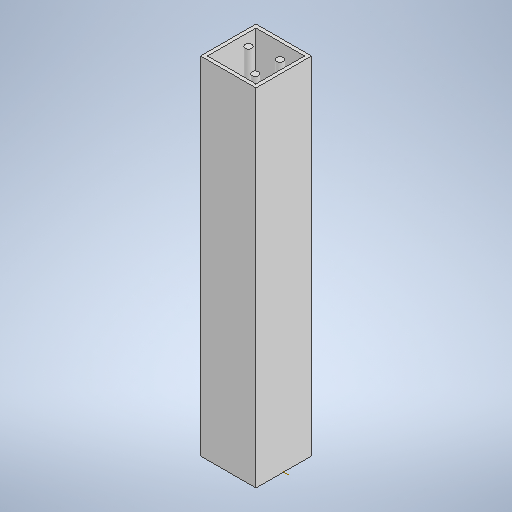
# Autodesk Inventor part: TS_Magazin_int
Saved by Autodesk Inventor 2025.2 (Build 292293000, 293)
## iProperties
Created: 2025-05-27
Part Number: TS_Magazin_int
Material: Generisch
Document SubType Name: Modeling
Designer: tino
Density: 1 g/cm^3
Appearance: Vorgabe
Mass: 3200 g
Surface Area: 1728 cm^2
Volume: 3200 cm^3
Author: tino
Autodesk Inventor part; units mm, degrees
ref_plane "YZ Plane" through (0, 0, 0) normal (1, 0, 0) x (0, 1, 0)
ref_plane "XZ Plane" through (0, 0, 0) normal (0, 1, 0) x (-1, 0, 0)
ref_plane "XY Plane" through (0, 0, 0) normal (0, 0, 1) x (1, 0, 0)
sketch "Skizze1" plane through (0, 0, 0) normal (0, 0, 1) x (1, 0, 0)
  line L0 (-40, 40) -> (40, 40)
  line L1 (40, 40) -> (40, -40)
  line L2 (40, -40) -> (-40, -40)
  line L3 (-40, -40) -> (-40, 40)
  line L4 (-40, 40) -> (40, -40) construction
  line L5 (40, 40) -> (-40, -40) construction
  point P0 (0, 0)
  dimension "d0" = 80
  dimension "d1" = 80
  constraints: 12 end point, 2 midpoint, 2 parallel, 1 horizontal, 1 perpendicular
  measures "d0" distance of L0.start L0.end
  measures "d1" distance of L0.end L1.end
extrude "Extrusion1" add sketch "Skizze1" along normal blind 500
sketch "Skizze2" plane through (0, 0, 500) normal (0, 0, 1) x (1, 0, 0)
  spline S0 degree 3 poles (30.8941, -22.3608) (33.2455, -20.1357) (33.4278, -16.4642) (34.1009, -12.3897) (34.4408, -6.5615) (32.3239, 0.3889) (27.6464, 2.5629) (18.7777, 8.3578) (6.0522, 19.3642) (-10.5837, 24.0919) (-22.9305, 22.7109) (-28.1368, 17.5955) (-28.9312, 16.6042) knots 0 0 0 0 0.05535 0.076528 0.211782 0.295547 0.382964 0.432922 0.754884 0.81234 0.967238 1 1 1 1
  spline S1 degree 3 poles (-28.9312, 16.6042) (-32.363, 12.3217) (-33.9219, 4.96) (-34.2212, -5.2183) (-33.7128, -11.7973) (-30.1787, -16.4552) (-26.4199, -18.3019) (-21.7499, -13.8164) (-22.8916, -9.4321) (-23.5075, -1.7153) (-24.1566, 7.4043) (-16.6489, 14.0721) (-3.6681, 12.4997) (3.1986, 4.5284) (3.2907, 1.6248) (4.5253, 0.0908) (6.4773, -0.7371) (8.3789, 1.0012) (13.1845, -1.0041) (13.637, -9.218) (17.043, -16.25) (23.183, -17.8067) (25.3482, -18.6227) (26.133, -19.8789) (26.5745, -22.0212) (27.7048, -23.641) (30.0236, -23.1574) (30.8172, -22.4336) (30.8941, -22.3608) knots 0 0 0 0 0.14153 0.17035 0.245987 0.25892 0.290227 0.326265 0.372233 0.38898 0.482096 0.508256 0.624416 0.647418 0.715274 0.72607 0.746892 0.801722 0.811885 0.848514 0.916356 0.943374 0.948219 0.962959 0.96651 0.98188 0.998188 1 1 1 1
  arc A0 (27.4787, -6.7498) -> (23.9934, -5.2356) centre (25, -7.687) ccw
  line L0 (27.4787, -6.7498) -> (26.0066, -10.1384)
  arc A1 (22.5213, -8.6242) -> (26.0066, -10.1384) centre (25, -7.687) ccw
  line L1 (22.5213, -8.6242) -> (23.9934, -5.2356)
  line L2 (22.5213, -8.6242) -> (23.9934, -5.2356)
  arc A2 (22.5213, -8.6242) -> (26.0066, -10.1384) centre (25, -7.687) ccw
  line L3 (27.4787, -6.7498) -> (26.0066, -10.1384)
  arc A3 (27.4787, -6.7498) -> (23.9934, -5.2356) centre (25, -7.687) ccw
  line L4 (-40, 40) -> (-40, -40) construction
  line L5 (-40, 0) -> (40, 0) construction
  line L6 (40, -40) -> (40, 40) construction
  line L7 (-34.1215, 23.4036) -> (-34.1215, -17.2519) construction
  line L8 (34.1216, 27.1841) -> (34.1216, -29.8621) construction
  line L9 (-36.6715, 23.259) -> (37.4151, 23.259) construction
  line L10 (-34.1215, -23.2592) -> (37.4151, -23.2592) construction
  point P0 (0, 0)
  point P1 (0, 0)
  dimension "d4" = 34.1215
  dimension "d6" = 34.1216
  dimension "d10" = 23.259
  dimension "d11" = 23.2592
  constraints: 18 end point, 8 point on circle, 4 centre point, 4 vertical, 3 midpoint, 2 horizontal, 2 perpendicular, 4 other
  measures "d4" distance from line of L7 point (0, 0)
  measures "d6" distance from line of L8 point (0, 0)
  measures "d10" distance from line of point (0, 0) L9
  measures "d11" distance from line of point (0, 0) L10
extrude "Extrusion2" cut sketch "Skizze2" against normal blind 500 contours S1 S0 | L0 A1 L1 A0
sketch "Skizze4" plane through (0, 0, 500) normal (0, 0, 1) x (1, 0, 0)
  circle A0 centre (-17.4445, 6.5749) radius 5
  circle A1 centre (21.6177, 12.9178) radius 5
  circle A2 centre (21.6177, -22.6069) radius 5
  point P0 (0, 0)
  dimension "d14" = 10
  dimension "d15" = 10
  dimension "d16" = 10
  dimension "d17" = 6.5749
  constraints: 3 centre point, 1 vertical alignment, 6 other
  measures "d14" diameter of A0
  measures "d15" diameter of A1
  measures "d16" diameter of A2
  measures "d17" vertical distance of point (0, 0) A0.centre
sketch "Skizze5" plane through (0, 0, 500) normal (0, 0, 1) x (1, 0, 0)
  line L0 (-35, 35) -> (35, 35)
  line L1 (35, 35) -> (35, -35)
  line L2 (35, -35) -> (-35, -35)
  line L3 (-35, -35) -> (-35, 35)
  line L4 (-35, 35) -> (35, -35) construction
  line L5 (35, 35) -> (-35, -35) construction
  spline S0 degree 3 poles (-28.9312, 16.6042) (-28.1368, 17.5955) (-22.9305, 22.7109) (-10.5837, 24.0919) (6.0522, 19.3642) (18.7777, 8.3578) (27.6464, 2.5629) (32.3239, 0.3889) (34.4408, -6.5615) (34.1009, -12.3897) (33.4278, -16.4642) (33.2455, -20.1357) (30.8941, -22.3608) knots 0 0 0 0 0.032762 0.18766 0.245116 0.567078 0.617036 0.704453 0.788218 0.923472 0.94465 1 1 1 1
  spline S1 degree 3 poles (30.8941, -22.3608) (30.8172, -22.4336) (30.0236, -23.1574) (27.7048, -23.641) (26.5745, -22.0212) (26.133, -19.8789) (25.3482, -18.6227) (23.183, -17.8067) (17.043, -16.25) (13.637, -9.218) (13.1845, -1.0041) (8.3789, 1.0012) (6.4773, -0.7371) (4.5253, 0.0908) (3.2907, 1.6248) (3.1986, 4.5284) (-3.6681, 12.4997) (-16.6489, 14.0721) (-24.1566, 7.4043) (-23.5075, -1.7153) (-22.8916, -9.4321) (-21.7499, -13.8164) (-26.4199, -18.3019) (-30.1787, -16.4552) (-33.7128, -11.7973) (-34.2212, -5.2183) (-33.9219, 4.96) (-32.363, 12.3217) (-28.9312, 16.6042) knots 0 0 0 0 0.001812 0.01812 0.03349 0.037041 0.051781 0.056626 0.083644 0.151486 0.188115 0.198278 0.253108 0.27393 0.284726 0.352582 0.375584 0.491744 0.517904 0.61102 0.627767 0.673735 0.709773 0.74108 0.754013 0.82965 0.85847 1 1 1 1
  point P0 (0, 0)
  dimension "d18" = 70
  dimension "d19" = 70
  constraints: 12 end point, 2 midpoint, 2 parallel, 1 horizontal, 1 perpendicular
  measures "d18" distance of L0.start L0.end
  measures "d19" distance of L0.end L1.end
extrude "Extrusion3" cut sketch "Skizze5" against normal blind 500
extrude "Extrusion4" add sketch "Skizze4" against normal blind 500
equation "\"d0\" = Magazin_Laenge"
equation "\"d1\" = Magazin_Breite"
equation "\"d2\" = Magazin_Hoehe"
equation "\"d12\" = Magazin_Hoehe"
equation "\"d18\" = Magazin_Breite - 2 * Wanddicke"
equation "\"d19\" = Magazin_Laenge - 2 * Wanddicke"
equation "\"d20\" = Magazin_Hoehe"
equation "\"d22\" = Magazin_Hoehe"
equation "\"Magazin_Breite\" = 80"
equation "\"Magazin_Hoehe\" = 500"
equation "\"Magazin_Laenge\" = 80"
equation "\"Wanddicke\" = 5"
